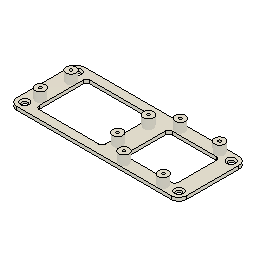
esu-bridge-bracket (Autodesk Fusion 360 design; units mm, degrees)
Autodesk Fusion 360 part; units mm, degrees
note: some values were not read from the file. Set by a fixed rule: the direction of a hole.
sketch "esu-bridge-bracket" plane through (0, 0, 0) normal (0, 1, 0) x (1, 0, 0)
  circle A0 centre (121.158, 44.958) radius 3.302
  circle A1 centre (121.158, 5.842) radius 3.302
  line L0 (13.462, 6.35) -> (13.462, 44.45)
  circle A2 centre (5.842, 44.958) radius 2.159
  circle A3 centre (81.534, 46.482) radius 3.81
  line L1 (13.462, 6.35) -> (63.2219, 6.35)
  line L2 (77.216, 8.636) -> (115.316, 8.636)
  arc A4 (0, 5.842) -> (5.842, 0) centre (5.842, 5.842) ccw
  arc A5 (5.842, 50.8) -> (0, 44.958) centre (5.842, 44.958) ccw
  arc A6 (121.158, 0) -> (127, 5.842) centre (121.158, 5.842) ccw
  line L3 (13.462, 44.45) -> (63.2219, 44.45)
  line L4 (127, 5.842) -> (127, 44.958)
  line L5 (63.2219, 6.35) -> (63.2219, 44.45)
  circle A7 centre (5.842, 5.842) radius 2.159
  circle A8 centre (121.158, 44.958) radius 2.159
  circle A9 centre (110.998, 4.318) radius 1.143
  arc A10 (127, 44.958) -> (121.158, 50.8) centre (121.158, 44.958) ccw
  line L6 (0, 5.842) -> (0, 44.958)
  circle A11 centre (110.998, 46.482) radius 3.81
  line L7 (115.316, 42.164) -> (115.316, 8.636)
  circle A12 centre (67.3419, 36.9) radius 3.81
  circle A13 centre (67.3419, 36.9) radius 1.143
  circle A14 centre (121.158, 5.842) radius 2.159
  circle A15 centre (5.842, 5.842) radius 3.302
  line L8 (5.842, 50.8) -> (121.158, 50.8)
  circle A16 centre (5.842, 44.958) radius 3.302
  line L9 (77.216, 42.164) -> (115.316, 42.164)
  circle A17 centre (81.534, 46.482) radius 1.143
  line L10 (77.216, 42.164) -> (77.216, 8.636)
  circle A18 centre (9.342, 36.9) radius 3.81
  circle A19 centre (81.534, 4.318) radius 3.81
  circle A20 centre (9.342, 13.9) radius 1.143
  circle A21 centre (9.342, 36.9) radius 1.143
  circle A22 centre (81.534, 4.318) radius 1.143
  circle A23 centre (67.3419, 13.9) radius 3.81
  circle A24 centre (110.998, 46.482) radius 1.143
  line L11 (5.842, 0) -> (121.158, 0)
  circle A25 centre (67.3419, 13.9) radius 1.143
  circle A26 centre (9.342, 13.9) radius 3.81
  circle A27 centre (110.998, 4.318) radius 3.81
extrude "Extrude5" add sketch "esu-bridge-bracket" along normal blind 2.54 contours A0 | A1 | A2 | A3 | A4 A5 A6 L4 A10 L6 L8 L11 | A7 | A8 | A9 | A11 | A12 | A13 | A14 | A15 | A16 | A17 | A18 | A19 | A20 | A21 | A22 | A23 | A24 | A25 | A26 | A27 makes body 1
extrude "Extrude7" add sketch "esu-bridge-bracket" along normal blind 9.525 separate body contours A3 | A9 | A11 | A12 | A13 | A17 | A18 | A19 | A20 | A21 | A22 | A23 | A24 | A25 | A26 | A27 makes body 2 at (85.3393, 6.35, -4.1281) makes body 3 at (13.1473, 6.35, -13.7101) makes body 4 at (69.8629, 6.35, -16.7567) makes body 5 at (114.8033, 6.35, -4.1281) makes body 6 at (85.3393, 6.35, -46.2921) makes body 7 at (13.1473, 6.35, -36.7101) makes body 8 at (71.1471, 6.35, -36.7101) makes body 9 at (108.3377, 6.35, -49.2095)
hole "Hole1" at (5.842, 0, -44.958) at (5.842, 0, -5.842) at (121.158, 0, -5.842) at (121.158, 0, -44.958) direction (0, 1, 0) diameter 4.318 depth 2.54 tip angle 118 bodies 1
fillet "Fillet1" radius 2.54 4 edges at (13.462, 1.27, -44.45) (13.462, 1.27, -6.35) (63.2219, 1.27, -6.35) (63.2219, 1.27, -44.45) on bodies 1
fillet "Fillet2" radius 2.54 4 edges at (115.316, 1.27, -8.636) (115.316, 1.27, -42.164) (77.216, 1.27, -42.164) (77.216, 1.27, -8.636) on bodies 1
hole "Hole2" at (9.342, 0, -13.9) at (9.342, 0, -36.9) at (67.3419, 0, -36.9) at (67.3419, 0, -13.9) at (81.534, 0, -4.318) at (110.998, 0, -4.318) at (110.998, 0, -46.482) at (81.534, 0, -46.482) direction (0, 1, 0) diameter 2.032 depth 9.525 tip angle 180 bodies 2 8 6 9 7 5 3 4
chamfer "Chamfer1" distance 1.143 angle 45 4 edges at (5.0613, 2.54, -3.8291) (120.3773, 2.54, -3.8291) (120.3773, 2.54, -42.9451) (5.0613, 2.54, -42.9451) on bodies 1
